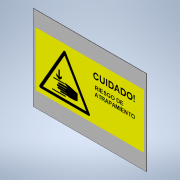
# Autodesk Inventor part: Advertencia
Saved by Autodesk Inventor 2021 (Build 250183000, 183)
## iProperties
Created: 2021-07-11
Part Number: Advertencia
Material: Generic
Document SubType Name: Modeling
Designer: Nelson
Density: 1 g/cm^3
Appearance: Default
Author: Nelson
Autodesk Inventor part; units mm, degrees
ref_plane "YZ Plane" through (0, 0, 0) normal (1, 0, 0) x (0, 1, 0)
ref_plane "XZ Plane" through (0, 0, 0) normal (0, 1, 0) x (-1, 0, 0)
ref_plane "XY Plane" through (0, 0, 0) normal (0, 0, 1) x (1, 0, 0)
sketch "Sketch1" plane through (0, 0, 0) normal (0, 0, 1) x (1, 0, 0)
  line L0 (0, 0) -> (400, 0)
  line L1 (400, 0) -> (400, 300)
  line L2 (400, 300) -> (0, 300)
  line L3 (0, 300) -> (0, 0)
  dimension "d0" = 400
  dimension "d1" = 300
  constraints: 8 end point, 2 parallel, 1 horizontal, 1 perpendicular
  measures "d0" distance of L2.end L1.end
  measures "d1" distance of L1.end L0.end
extrude "Extrusion1" add sketch "Sketch1" along normal blind 0.9
sketch "Sketch2" plane through (0, 0, 0.9) normal (0, 0, 1) x (1, 0, 0)
  line L0 (8.52, 246.5646) -> (391.4673, 246.5646) construction
  line L1 (391.4673, 246.5646) -> (391.4673, 53.4355) construction
  line L2 (391.4673, 53.4355) -> (8.52, 53.4355) construction
  line L3 (8.52, 53.4355) -> (8.52, 246.5646) construction
  line L4 (0, 0) -> (400, 0) projected
  line L5 (0, 300) -> (0, 0) projected
  dimension "d40" = 53.4355
  dimension "d41" = 8.52
  constraints: 2 other
  measures "d40" distance between parallel lines of L4 L2
  measures "d41" distance between parallel lines of L3 L5
decal "Decal1"
body "Solid1"
